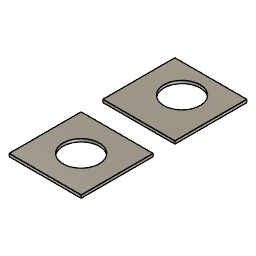
Oct26_Design_Intent_Exercise (Autodesk Fusion 360 design; units mm, degrees)
part number: 2025-10-26-14-24-35-716
part number: 2025-10-26-14-30-05-261
part number: 2025-10-26-14-45-48-401
Autodesk Fusion 360 part; units mm, degrees
sketch "Sketch1" plane through (0, 0, 0) normal (0, 0, 1) x (1, 0, 0) in component "Plate1"
  line L0 (-50, 50) -> (50, 50)
  line L1 (50, 50) -> (50, -50)
  line L2 (50, -50) -> (-50, -50)
  line L3 (-50, -50) -> (-50, 50)
  line L4 (-50, 50) -> (50, -50) construction
  line L5 (50, 50) -> (-50, -50) construction
  circle A0 centre (0, 0) radius 25
  dimension "d5" = 100
  dimension "d6" = 50
  constraint horizontal L0
  constraint perpendicular L0 L1
  constraint parallel L0 L2
  constraint parallel L1 L3
  constraint coincident L4 A0.centre
  constraint coincident L5 A0.centre
  constraint coincident A0.centre origin
  constraint equal L1 L2
  measures "d5" distance of L0.end L1.end
  measures "d6" diameter of A0
extrude "Extrude1" add sketch "Sketch1" along normal blind 4 makes body 1 in component "Plate1"
sketch "Sketch1 (2)" plane through (0, 0, 0) normal (0, 0, 1) x (1, 0, 0) in component "Plate1 (1)"
  line L0 (-50, 50) -> (50, 50)
  line L1 (50, 50) -> (50, -50)
  line L2 (50, -50) -> (-50, -50)
  line L3 (-50, -50) -> (-50, 50)
  line L4 (-50, 50) -> (50, -50) construction
  line L5 (50, 50) -> (-50, -50) construction
  circle A0 centre (0, 10) radius 25
  dimension "d5_1" = 100
  dimension "d6_1" = 50
  dimension "d9" = 40
  constraint horizontal L0
  constraint perpendicular L0 L1
  constraint parallel L0 L2
  constraint parallel L1 L3
  constraint coincident L4 origin
  constraint coincident L5 origin
  constraint equal L1 L2
  constraint vertical origin A0.centre
  measures "d5_1" distance of L0.end L1.end
  measures "d6_1" diameter of A0
  measures "d9" distance of L0 A0.centre
extrude "Extrude1'" add sketch "Sketch1 (2)" along normal blind 4 separate body makes body 2 in component "Plate1 (1)"
component "Plate1" placed x (1, 0, 0) y (0, 1, 0) z (0, 0, 1) at (0, 0, 0)
component "Plate1 (1)" placed x (1, 0, 0) y (0, 1, 0) z (0, 0, 1) at (0, 0, 0)
equation "d6 = d5 / 2"
